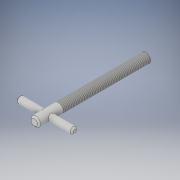
# Autodesk Inventor part: screw
Saved by Autodesk Inventor 2019.3 (Build 233278000, 278)
## iProperties
Created: 2019-04-14
Part Number: screw
Material: Generic
Document SubType Name: Modeling
Designer: peter
Density: 1 g/cm^3
Appearance: Default
Author: peter
Autodesk Inventor part; units mm, degrees
ref_plane "YZ Plane" through (0, 0, 0) normal (1, 0, 0) x (0, 1, 0)
ref_plane "XZ Plane" through (0, 0, 0) normal (0, 1, 0) x (-1, 0, 0)
ref_plane "XY Plane" through (0, 0, 0) normal (0, 0, 1) x (1, 0, 0)
sketch "Sketch1" plane through (0, 0, 0) normal (0, 0, 1) x (1, 0, 0)
  circle A0 centre (0, 0) radius 3
  dimension "d0" = 6
  constraints: 1 centre point, 1 coincident
  measures "d0" diameter of A0
extrude "Extrusion1" add sketch "Sketch1" along normal blind 70
thread "Thread1" size "M6x1" class "6g" standard "ANSI Metric M Profile" length 55
chamfer "Chamfer1" distance 1 angle 45 1 edges at (-3, 0, 70)
sketch "Sketch2" plane through (0, 0, 0) normal (1, 0, 0) x (0, 1, 0)
  line L0 (-2, 70) -> (2, 70) construction
  line L1 (0, 70) -> (0, 62) construction
  circle A0 centre (0, 62) radius 2
  point P0 (0, 0)
  dimension "d8" = 8
  dimension "d9" = 4
  constraints: 2 end point, 1 centre point, 1 coincident, 1 midpoint, 1 vertical
  measures "d8" distance of L1.start L1.end
  measures "d9" diameter of A0
extrude "Extrusion2" add sketch "Sketch2" along normal mid plane 35
chamfer "Chamfer2" distance 1 angle 45 2 edges at (17.5, -2, 62) (-17.5, -2, 62)
body "Solid1"
